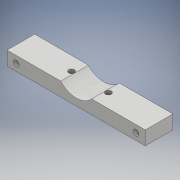
# Autodesk Inventor part: side_humidity_support
Saved by Autodesk Inventor 2017 (Build 210142000, 142)
## iProperties
Created: 2018-03-12
Part Number: side_humidity_support
Material: Generic
Document SubType Name: Modeling
Designer: Nic
Density: 1 g/cm^3
Appearance: Default
Author: Nic
Autodesk Inventor part; units mm, degrees
ref_plane "YZ Plane" through (0, 0, 0) normal (1, 0, 0) x (0, 1, 0)
ref_plane "XZ Plane" through (0, 0, 0) normal (0, 1, 0) x (-1, 0, 0)
ref_plane "XY Plane" through (0, 0, 0) normal (0, 0, 1) x (1, 0, 0)
sketch "Sketch1" plane through (0, 0, 0) normal (0, 0, 1) x (1, 0, 0)
  line L0 (-30, 6) -> (30, 6)
  line L1 (30, 6) -> (30, -6)
  line L2 (30, -6) -> (-30, -6)
  line L3 (-30, -6) -> (-30, 6)
  line L4 (0, 0) -> (0, 6) construction
  line L5 (0, 0) -> (30, 0) construction
  circle A0 centre (-8, 0) radius 1.25
  circle A1 centre (8, 0) radius 1.25
  dimension "d0" = 12
  dimension "d1" = 60
  dimension "d2" = 16
  dimension "d3" = 2.5
  constraints: 12 end point, 3 perpendicular, 2 centre point, 2 midpoint, 2 parallel, 1 horizontal, 1 point on line, 3 other
  measures "d0" distance of L0.end L1.end
  measures "d1" distance of L1.end L2.end
  measures "d2" distance of A1.centre A0.centre
  measures "d3" diameter of A0
extrude "Extrusion1" add sketch "Sketch1" along normal blind 6
sketch "Sketch2" plane through (-30, 6, 0) normal (0, 1, 0) x (1, 0, 0)
  circle A0 centre (4, -3) radius 1.25
  circle A1 centre (56, -3) radius 1.25
  arc A2 (38.4853, -9) -> (21.5147, -9) centre (30, -12) ccw
  line L0 (0, 0) -> (0, -6) projected
  line L1 (30, 0) -> (30, -6) construction
  line L2 (60, -6) -> (0, -6) projected
  line L3 (4, -3) -> (56, -3) construction
  line L4 (0, 0) -> (60, 0) construction
  line L5 (21.5147, -9) -> (38.4853, -9)
  dimension "d6" = 4
  dimension "d7" = 2.5
  dimension "d8" = 3
  dimension "d9" = 18
  dimension "d10" = 3
  constraints: 6 end point, 3 centre point, 2 midpoint, 2 point on circle, 1 horizontal, 1 parallel, 1 tangent, 1 vertical alignment, 1 other
  measures "d6" distance from line of L0 L3.start
  measures "d7" diameter of A0
  measures "d8" distance between parallel lines of L2 L3
  measures "d9" diameter of A2
  measures "d10" distance between parallel lines of L2 L5
extrude "Extrusion2" cut sketch "Sketch2" against normal up to next
body "Solid1"
